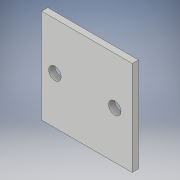
# Autodesk Inventor part: Buste3
Saved by Autodesk Inventor 2018 (Build 220112000, 112)
## iProperties
Created: 2018-02-13
Part Number: Buste3
Material: Generic
Document SubType Name: Modeling
Designer: Lilia
Density: 1 g/cm^3
Appearance: Default
Author: Lilia
Autodesk Inventor part; units mm, degrees
ref_plane "YZ Plane" through (0, 0, 0) normal (1, 0, 0) x (0, 1, 0)
ref_plane "XZ Plane" through (0, 0, 0) normal (0, 1, 0) x (-1, 0, 0)
ref_plane "XY Plane" through (0, 0, 0) normal (0, 0, 1) x (1, 0, 0)
sketch "Sketch1" plane through (0, 0, 0) normal (0, 0, 1) x (1, 0, 0)
  line L0 (-47.45, 49.4) -> (47.45, 49.4)
  line L1 (47.45, 49.4) -> (47.45, -49.4)
  line L2 (47.45, -49.4) -> (-47.45, -49.4)
  line L3 (-47.45, -49.4) -> (-47.45, 49.4)
  line L4 (-47.45, 49.4) -> (47.45, -49.4) construction
  line L5 (47.45, 49.4) -> (-47.45, -49.4) construction
  point P0 (0, 0)
  dimension "Comp" = 94.9
  dimension "Larg" = 98.8
  constraints: 12 end point, 2 midpoint, 2 parallel, 1 horizontal, 1 perpendicular
  measures "Comp" distance of L0.start L0.end
  measures "Larg" distance of L2.end L0.start
extrude "Extrusion1" add sketch "Sketch1" along normal mid plane 6.5
hole "Hole2" at (-33.45, 0, 3.25) direction (0, 0, -1) diameter 13 end through all
hole "Hole3" at (29.25, 0, 3.25) direction (0, 0, -1) diameter 13 end through all
body "Solid1"
